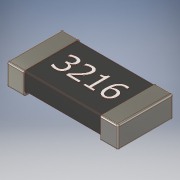
# Autodesk Inventor part: Resistor_3216-0.65mm
Saved by Autodesk Inventor 2018 (Build 220112000, 112)
## iProperties
Created: 2016-08-15
Part Number: Resistor_3216-0.65mm
Material: Copper
Document SubType Name: Modeling
Designer: Bradley
Density: 8.94 g/cm^3
Appearance: Copper - Satin
Author: Bradley
Autodesk Inventor part; units mm, degrees
ref_plane "YZ Plane" through (0, 0, 0) normal (1, 0, 0) x (0, 1, 0)
ref_plane "XZ Plane" through (0, 0, 0) normal (0, 1, 0) x (-1, 0, 0)
ref_plane "XY Plane" through (0, 0, 0) normal (0, 0, 1) x (1, 0, 0)
sketch "Sketch1" plane through (0, 0, 0) normal (0, 0, 1) x (1, 0, 0)
  line L0 (-1.6, 0.535) -> (-1.1, 0.535)
  line L1 (-1.1, 0.535) -> (-1.1, -0.1)
  line L2 (-1.1, -0.1) -> (-1.6, -0.1)
  line L3 (-1.6, -0.1) -> (-1.6, 0.535)
  line L4 (-1.1, 0.525) -> (1.1, 0.525)
  line L5 (1.1, 0.525) -> (1.1, 0)
  line L6 (1.1, 0) -> (-1.1, 0)
  line L7 (-1.1, 0) -> (-1.1, 0.525)
  line L8 (1.1, 0.535) -> (1.6, 0.535)
  line L9 (1.6, 0.535) -> (1.6, -0.1)
  line L10 (1.6, -0.1) -> (1.1, -0.1)
  line L11 (1.1, -0.1) -> (1.1, 0.535)
  point P0 (0, 0)
  point P1 (0, 0.525)
  point P2 (0, 0)
  dimension "d0" = 3.2
  dimension "d1" = 0.635
  dimension "d2" = 0.5
  dimension "d3" = 0.1
  dimension "d6" = 0.01
  constraints: 24 end point, 6 parallel, 3 horizontal, 3 perpendicular, 3 point on line, 2 collinear, 2 midpoint, 1 coincident, 1 vertical alignment
  measures "d0" distance between parallel lines of L9 L3
  measures "d1" distance of L2.end L0.start
  measures "d2" distance of L1.end L2.end
  measures "d3" distance between parallel lines of L2 L6
  measures "d6" distance between parallel lines of L4 L0
extrude "Extrusion1" add sketch "Sketch1" along normal mid plane 1.6 contours L0 L1 L2 L3 | L11 L8 L9 L10 L5
extrude "Extrusion2" add sketch "Sketch1" along normal mid plane 1.55 contours L4 L5 L6 L1
sketch "Sketch3" plane through (-1.1, 0.525, 0.775) normal (0, 1, 0) x (1, 0, 0)
  line L0 (0, 0) -> (0, 1.55) projected
  line L1 (2.2, 0) -> (0, 0) projected
  line L2 (2.2, 1.55) -> (2.2, 0) projected
  line L3 (0, 1.55) -> (2.2, 1.55) projected
  line L4 (2.2, 1.575) -> (2.2, -0.025) construction
  line L5 (2.2, 0.4859) -> (0, 0.4859) construction
  line L6 (0, 1.575) -> (0, -0.025) construction
  spline S0 degree 2 poles (0.4052, 1.029) (0.3833, 1.029) (0.34, 1.0183) (0.3191, 1.0101) knots 0 0 0 1 2 2 2
  spline S1 degree 2 poles (0.3191, 1.0101) (0.2997, 1.0018) (0.271, 0.9843) (0.2598, 0.9765) knots 0 0 0 1 2 2 2
  line L7 (0.2598, 0.9765) -> (0.2549, 0.9765)
  line L8 (0.2549, 0.9765) -> (0.2549, 1.0616)
  spline S2 degree 2 poles (0.2549, 1.0616) (0.2812, 1.0757) (0.3712, 1.0985) (0.4115, 1.0985) knots 0 0 0 1 2 2 2
  spline S3 degree 2 poles (0.4115, 1.0985) (0.4524, 1.0985) (0.5131, 1.082) (0.5379, 1.0645) knots 0 0 0 1 2 2 2
  spline S4 degree 2 poles (0.5379, 1.0645) (0.5642, 1.0455) (0.5914, 0.9906) (0.5914, 0.9537) knots 0 0 0 1 2 2 2
  spline S5 degree 2 poles (0.5914, 0.9537) (0.5914, 0.9041) (0.5263, 0.8292) (0.4806, 0.8195) knots 0 0 0 1 2 2 2
  line L9 (0.4806, 0.8195) -> (0.4806, 0.8136)
  spline S6 degree 2 poles (0.4806, 0.8136) (0.4995, 0.8097) (0.5428, 0.7922) (0.5613, 0.7747) knots 0 0 0 1 2 2 2
  spline S7 degree 2 poles (0.5613, 0.7747) (0.5797, 0.7577) (0.6031, 0.7032) (0.6031, 0.6639) knots 0 0 0 1 2 2 2
  spline S8 degree 2 poles (0.6031, 0.6639) (0.6031, 0.6235) (0.5754, 0.5549) (0.5501, 0.5287) knots 0 0 0 1 2 2 2
  spline S9 degree 2 poles (0.5501, 0.5287) (0.5238, 0.5015) (0.4494, 0.4733) (0.4023, 0.4733) knots 0 0 0 1 2 2 2
  spline S10 degree 2 poles (0.4023, 0.4733) (0.3571, 0.4733) (0.2686, 0.4951) (0.2384, 0.5102) knots 0 0 0 1 2 2 2
  line L10 (0.2384, 0.5102) -> (0.2384, 0.5953)
  line L11 (0.2384, 0.5953) -> (0.2442, 0.5953)
  spline S11 degree 2 poles (0.2442, 0.5953) (0.2695, 0.5768) (0.3551, 0.5428) (0.3974, 0.5428) knots 0 0 0 1 2 2 2
  spline S12 degree 2 poles (0.3974, 0.5428) (0.4222, 0.5428) (0.4718, 0.5584) (0.4883, 0.5763) knots 0 0 0 1 2 2 2
  spline S13 degree 2 poles (0.4883, 0.5763) (0.5044, 0.5943) (0.5214, 0.6371) (0.5214, 0.6697) knots 0 0 0 1 2 2 2
  spline S14 degree 2 poles (0.5214, 0.6697) (0.5214, 0.7023) (0.5024, 0.7446) (0.4854, 0.7567) knots 0 0 0 1 2 2 2
  spline S15 degree 2 poles (0.4854, 0.7567) (0.4684, 0.7689) (0.4222, 0.7781) (0.395, 0.7781) knots 0 0 0 1 2 2 2
  line L12 (0.395, 0.7781) -> (0.3609, 0.7781)
  line L13 (0.3609, 0.7781) -> (0.3609, 0.8447)
  line L14 (0.3609, 0.8447) -> (0.3877, 0.8447)
  spline S16 degree 2 poles (0.3877, 0.8447) (0.4417, 0.8447) (0.5097, 0.8963) (0.5097, 0.9454) knots 0 0 0 1 2 2 2
  spline S17 degree 2 poles (0.5097, 0.9454) (0.5097, 0.9682) (0.4922, 1.0008) (0.4781, 1.0105) knots 0 0 0 1 2 2 2
  spline S18 degree 2 poles (0.4781, 1.0105) (0.463, 1.0208) (0.4261, 1.029) (0.4052, 1.029) knots 0 0 0 1 2 2 2
  line L15 (1.0635, 0.4859) -> (0.6935, 0.4859)
  line L16 (0.6935, 0.4859) -> (0.6935, 0.571)
  spline S19 degree 2 poles (0.6935, 0.571) (0.7334, 0.6084) (0.8044, 0.678) (0.8384, 0.7154) knots 0 0 0 1 2 2 2
  spline S20 degree 2 poles (0.8384, 0.7154) (0.907, 0.7908) (0.9571, 0.8812) (0.9571, 0.9293) knots 0 0 0 1 2 2 2
  spline S21 degree 2 poles (0.9571, 0.9293) (0.9571, 0.9546) (0.9415, 0.9925) (0.9274, 1.0047) knots 0 0 0 1 2 2 2
  spline S22 degree 2 poles (0.9274, 1.0047) (0.9133, 1.0169) (0.8763, 1.029) (0.854, 1.029) knots 0 0 0 1 2 2 2
  spline S23 degree 2 poles (0.854, 1.029) (0.8326, 1.029) (0.7888, 1.0183) (0.7689, 1.0101) knots 0 0 0 1 2 2 2
  spline S24 degree 2 poles (0.7689, 1.0101) (0.7519, 1.0032) (0.7203, 0.9838) (0.7105, 0.977) knots 0 0 0 1 2 2 2
  line L17 (0.7105, 0.977) -> (0.7062, 0.977)
  line L18 (0.7062, 0.977) -> (0.7062, 1.0626)
  spline S25 degree 2 poles (0.7062, 1.0626) (0.731, 1.0747) (0.8199, 1.0985) (0.8598, 1.0985) knots 0 0 0 1 2 2 2
  spline S26 degree 2 poles (0.8598, 1.0985) (0.9439, 1.0985) (1.0387, 1.0096) (1.0387, 0.9337) knots 0 0 0 1 2 2 2
  spline S27 degree 2 poles (1.0387, 0.9337) (1.0387, 0.8982) (1.0222, 0.8389) (1.0076, 0.8136) knots 0 0 0 1 2 2 2
  spline S28 degree 2 poles (1.0076, 0.8136) (0.993, 0.7874) (0.9507, 0.7358) (0.9274, 0.711) knots 0 0 0 1 2 2 2
  spline S29 degree 2 poles (0.9274, 0.711) (0.8895, 0.6697) (0.7966, 0.5812) (0.7689, 0.5554) knots 0 0 0 1 2 2 2
  line L19 (0.7689, 0.5554) -> (1.0635, 0.5554)
  line L20 (1.0635, 0.5554) -> (1.0635, 0.4859)
  line L21 (1.4836, 0.4859) -> (1.1909, 0.4859)
  line L22 (1.1909, 0.4859) -> (1.1909, 0.5472)
  line L23 (1.1909, 0.5472) -> (1.2998, 0.5472)
  line L24 (1.2998, 0.5472) -> (1.2998, 0.9493)
  line L25 (1.2998, 0.9493) -> (1.1909, 0.9493)
  line L26 (1.1909, 0.9493) -> (1.1909, 1.0042)
  spline S30 degree 2 poles (1.1909, 1.0042) (1.2527, 1.0042) (1.311, 1.0392) (1.3149, 1.0878) knots 0 0 0 1 2 2 2
  line L27 (1.3149, 1.0878) -> (1.3771, 1.0878)
  line L28 (1.3771, 1.0878) -> (1.3771, 0.5472)
  line L29 (1.3771, 0.5472) -> (1.4836, 0.5472)
  line L30 (1.4836, 0.5472) -> (1.4836, 0.4859)
  spline S31 degree 2 poles (1.9733, 0.6804) (1.9733, 0.6342) (1.9426, 0.5559) (1.9169, 0.5297) knots 0 0 0 1 2 2 2
  spline S32 degree 2 poles (1.9169, 0.5297) (1.8901, 0.5019) (1.823, 0.4733) (1.7827, 0.4733) knots 0 0 0 1 2 2 2
  spline S33 degree 2 poles (1.7827, 0.4733) (1.7423, 0.4733) (1.6757, 0.5005) (1.6504, 0.5277) knots 0 0 0 1 2 2 2
  spline S34 degree 2 poles (1.6504, 0.5277) (1.6193, 0.5603) (1.5843, 0.6697) (1.5843, 0.7494) knots 0 0 0 1 2 2 2
  spline S35 degree 2 poles (1.5843, 0.7494) (1.5843, 0.8277) (1.6164, 0.9537) (1.6499, 1.0003) knots 0 0 0 1 2 2 2
  spline S36 degree 2 poles (1.6499, 1.0003) (1.6825, 1.046) (1.7856, 1.0971) (1.8532, 1.0971) knots 0 0 0 1 2 2 2
  spline S37 degree 2 poles (1.8532, 1.0971) (1.8731, 1.0971) (1.9081, 1.0932) (1.9212, 1.0888) knots 0 0 0 1 2 2 2
  line L31 (1.9212, 1.0888) -> (1.9212, 1.0115)
  line L32 (1.9212, 1.0115) -> (1.9178, 1.0115)
  spline S38 degree 2 poles (1.9178, 1.0115) (1.9066, 1.0173) (1.8658, 1.0276) (1.8425, 1.0276) knots 0 0 0 1 2 2 2
  spline S39 degree 2 poles (1.8425, 1.0276) (1.7676, 1.0276) (1.6757, 0.9264) (1.6669, 0.8272) knots 0 0 0 1 2 2 2
  spline S40 degree 2 poles (1.6669, 0.8272) (1.6956, 0.8472) (1.7559, 0.869) (1.7919, 0.869) knots 0 0 0 1 2 2 2
  spline S41 degree 2 poles (1.7919, 0.869) (1.8269, 0.869) (1.8794, 0.8549) (1.9081, 0.8336) knots 0 0 0 1 2 2 2
  spline S42 degree 2 poles (1.9081, 0.8336) (1.9412, 0.8088) (1.9733, 0.7319) (1.9733, 0.6804) knots 0 0 0 1 2 2 2
  spline S43 degree 2 poles (1.8916, 0.677) (1.8916, 0.7139) (1.8721, 0.764) (1.8507, 0.7815) knots 0 0 0 1 2 2 2
  spline S44 degree 2 poles (1.8507, 0.7815) (1.8347, 0.7942) (1.7948, 0.8024) (1.7739, 0.8024) knots 0 0 0 1 2 2 2
  spline S45 degree 2 poles (1.7739, 0.8024) (1.7457, 0.8024) (1.6927, 0.7854) (1.6669, 0.7694) knots 0 0 0 1 2 2 2
  spline S46 degree 2 poles (1.6669, 0.7694) (1.6665, 0.7606) (1.6655, 0.7441) (1.6655, 0.7314) knots 0 0 0 1 2 2 2
  spline S47 degree 2 poles (1.6655, 0.7314) (1.6655, 0.6692) (1.6898, 0.5929) (1.7083, 0.5729) knots 0 0 0 1 2 2 2
  spline S48 degree 2 poles (1.7083, 0.5729) (1.7253, 0.554) (1.7622, 0.5389) (1.7831, 0.5389) knots 0 0 0 1 2 2 2
  spline S49 degree 2 poles (1.7831, 0.5389) (1.8318, 0.5389) (1.8916, 0.6079) (1.8916, 0.677) knots 0 0 0 1 2 2 2
  point P0 (1.1, 0.775)
  constraints: 2 end point, 2 point on line, 1 horizontal, 1 perpendicular
extrude "Extrusion4" add sketch "Sketch3" along normal blind 0.01 contours S0 S1 L7 L8 S2 S3 S4 S5 L9 S6 S7 S8 S9 S10 L10 L11 S11 S12 S13 S14 S15 L12 L13 L14 S16 S17 S18 | L15 L16 S19 S20 S21 S22 S23 S24 L17 L18 S25 S26 S27 S28 S29 L19 L20 | L21 L22 L23 L24 L25 L26 S30 L27 L28 L29 L30 | S31 S32 S33 S34 S35 S36 S37 L31 L32 S38 S39 S40 S41 S42
fillet "Fillet1" radius 0.05 22 edges at (-1.35, 0.535, 0.8) (0, 0.525, 0.775) (1.35, 0.535, 0.8) (-1.35, 0.535, -0.8) (0, 0.525, -0.775) (1.35, 0.535, -0.8) (1.6, 0.535, 0) (1.6, 0.2175, -0.8) (1.6, -0.1, 0) (1.35, -0.1, -0.8) (1.35, -0.1, 0.8) (1.6, 0.2175, 0.8) (0, 0, 0.775) (0, 0, -0.775) (-1.35, -0.1, -0.8) (-1.6, -0.1, 0) (-1.6, 0.2175, 0.8) (-1.35, -0.1, 0.8) (-1.6, 0.2175, -0.8) (-1.6, 0.535, 0) (-1.1, 0, 0) (1.1, 0, 0)
body "Solid1"
